Autodesk Inventor part; units mm, degrees
(part 2 of 2)
  spline S254 degree 2 poles (134.5802, -22.8415) (134.5802, -22.7633) (134.5214, -22.7045) (134.4921, -22.7045) knots 0 0 0 1 2 2 2
  spline S255 degree 2 poles (123.7465, -14.2784) (123.7074, -14.2784) (123.6487, -14.3273) (123.6487, -14.4154) knots 0 0 0 1 2 2 2
  line L195 (123.6487, -14.4154) -> (123.6487, -16.6761)
  spline S256 degree 2 poles (123.6487, -16.6761) (123.6487, -16.7544) (123.7074, -16.8229) (123.7465, -16.8229) knots 0 0 0 1 2 2 2
  spline S257 degree 2 poles (123.7465, -16.8229) (123.7759, -16.8229) (123.8346, -16.7641) (123.8346, -16.6761) knots 0 0 0 1 2 2 2
  line L196 (123.8346, -16.6761) -> (123.8346, -16.5391)
  spline S258 degree 2 poles (123.8346, -16.5391) (123.8248, -16.1476) (124.5001, -15.6191) (126.0855, -15.3647) (127.4458, -15.3647) knots 0 0 0 1 2 3 3 3
  line L197 (127.4458, -15.3647) -> (131.5366, -15.3647)
  spline S259 degree 2 poles (131.5366, -15.3647) (132.9262, -15.3451) (134.4627, -16.2944) (134.4725, -17.4981) knots 0 0 0 1 2 2 2
  spline S260 degree 2 poles (134.4725, -17.4981) (134.4529, -18.3398) (133.3764, -19.1325) (132.5054, -19.1227) knots 0 0 0 1 2 2 2
  line L198 (132.5054, -19.1227) -> (124.4414, -19.1227)
  spline S261 degree 2 poles (124.4414, -19.1227) (124.0695, -19.1325) (123.8248, -19.0738) (123.8346, -18.9661) knots 0 0 0 1 2 2 2
  line L199 (123.8346, -18.9661) -> (123.8346, -18.5061)
  spline S262 degree 2 poles (123.8346, -18.5061) (123.8346, -18.4181) (123.7759, -18.3593) (123.7465, -18.3691) knots 0 0 0 1 2 2 2
  spline S263 degree 2 poles (123.7465, -18.3691) (123.7074, -18.3691) (123.6487, -18.4278) (123.6487, -18.5061) knots 0 0 0 1 2 2 2
  line L200 (123.6487, -18.5061) -> (123.6487, -22.0391)
  spline S264 degree 2 poles (123.6487, -22.0391) (123.6487, -22.1173) (123.7074, -22.1761) (123.7465, -22.1761) knots 0 0 0 1 2 2 2
  spline S265 degree 2 poles (123.7465, -22.1761) (123.7759, -22.1761) (123.8346, -22.1173) (123.8346, -22.0391) knots 0 0 0 1 2 2 2
  line L201 (123.8346, -22.0391) -> (123.8346, -21.5987)
  spline S266 degree 2 poles (123.8346, -21.5987) (123.8248, -21.5008) (124.0695, -21.4323) (124.4414, -21.4323) knots 0 0 0 1 2 2 2
  line L202 (124.4414, -21.4323) -> (132.0944, -21.4323)
  spline S267 degree 2 poles (132.0944, -21.4323) (132.8088, -21.4323) (134.0223, -20.6787) (134.7563, -19.2206) (134.7661, -18.1538) knots 0 0 0 1 2 3 3 3
  spline S268 degree 2 poles (134.7661, -18.1538) (134.7759, -17.1556) (134.2083, -15.8246) (132.8382, -15.1592) (131.6442, -15.1592) knots 0 0 0 1 2 3 3 3
  line L203 (131.6442, -15.1592) -> (127.3382, -15.1592)
  spline S269 degree 2 poles (127.3382, -15.1592) (125.9778, -15.1592) (124.4414, -15.0222) (123.8248, -14.709) (123.8346, -14.4448) knots 0 0 0 1 2 3 3 3
  line L204 (123.8346, -14.4448) -> (123.8346, -14.4154)
  spline S270 degree 2 poles (123.8346, -14.4154) (123.8346, -14.3273) (123.7759, -14.2784) (123.7465, -14.2784) knots 0 0 0 1 2 2 2
  spline S271 degree 2 poles (134.4921, -4.4625) (134.4529, -4.4528) (134.3942, -4.5115) (134.3942, -4.5996) knots 0 0 0 1 2 2 2
  line L205 (134.3942, -4.5996) -> (134.3942, -5.0302)
  spline S272 degree 2 poles (134.3942, -5.0302) (134.404, -5.1378) (134.1691, -5.1867) (133.7972, -5.1867) knots 0 0 0 1 2 2 2
  line L206 (133.7972, -5.1867) -> (124.4414, -5.1867)
  spline S273 degree 2 poles (124.4414, -5.1867) (124.0695, -5.1867) (123.8248, -5.1378) (123.8346, -5.0302) knots 0 0 0 1 2 2 2
  line L207 (123.8346, -5.0302) -> (123.8346, -4.5996)
  spline S274 degree 2 poles (123.8346, -4.5996) (123.8346, -4.5115) (123.7759, -4.4528) (123.7465, -4.4625) knots 0 0 0 1 2 2 2
  spline S275 degree 2 poles (123.7465, -4.4625) (123.7074, -4.4625) (123.6487, -4.5213) (123.6487, -4.5996) knots 0 0 0 1 2 2 2
  line L208 (123.6487, -4.5996) -> (123.6487, -7.4866)
  spline S276 degree 2 poles (123.6487, -7.4866) (123.6487, -7.5746) (123.7172, -7.6431) (123.7759, -7.6431) knots 0 0 0 1 2 2 2
  line L209 (123.7759, -7.6431) -> (131.9182, -9.0035)
  line L210 (131.9182, -9.0035) -> (131.9182, -9.023)
  line L211 (131.9182, -9.023) -> (123.7759, -10.5497)
  spline S277 degree 2 poles (123.7759, -10.5497) (123.7172, -10.5693) (123.6487, -10.6574) (123.6487, -10.7259) knots 0 0 0 1 2 2 2
  line L212 (123.6487, -10.7259) -> (123.6487, -13.7303)
  spline S278 degree 2 poles (123.6487, -13.7303) (123.6487, -13.8086) (123.7074, -13.8576) (123.7465, -13.8478) knots 0 0 0 1 2 2 2
  spline S279 degree 2 poles (123.7465, -13.8478) (123.7759, -13.8576) (123.8346, -13.8086) (123.8346, -13.7303) knots 0 0 0 1 2 2 2
  line L213 (123.8346, -13.7303) -> (123.8346, -13.2312)
  spline S280 degree 2 poles (123.8346, -13.2312) (123.8248, -13.1334) (124.0695, -13.0746) (124.4414, -13.0746) knots 0 0 0 1 2 2 2
  line L214 (124.4414, -13.0746) -> (130.9004, -13.0746)
  spline S281 degree 2 poles (130.9004, -13.0746) (132.2608, -13.0746) (133.7972, -13.2117) (134.404, -13.5248) (134.3942, -13.7891) knots 0 0 0 1 2 3 3 3
  line L215 (134.3942, -13.7891) -> (134.3942, -13.8184)
  spline S282 degree 2 poles (134.3942, -13.8184) (134.3942, -13.9065) (134.4529, -13.9652) (134.4921, -13.9554) knots 0 0 0 1 2 2 2
  spline S283 degree 2 poles (134.4921, -13.9554) (134.5214, -13.9652) (134.5802, -13.8967) (134.5802, -13.8184) knots 0 0 0 1 2 2 2
  line L216 (134.5802, -13.8184) -> (134.5802, -11.7045)
  spline S284 degree 2 poles (134.5802, -11.7045) (134.5802, -11.6165) (134.5214, -11.5773) (134.4921, -11.5773) knots 0 0 0 1 2 2 2
  spline S285 degree 2 poles (134.4921, -11.5773) (134.4529, -11.5773) (134.3942, -11.6165) (134.3942, -11.7045) knots 0 0 0 1 2 2 2
  line L217 (134.3942, -11.7045) -> (134.3942, -11.8122)
  spline S286 degree 2 poles (134.3942, -11.8122) (134.404, -12.1645) (133.7874, -12.6343) (132.2118, -12.8593) (130.7928, -12.8593) knots 0 0 0 1 2 3 3 3
  line L218 (130.7928, -12.8593) -> (124.2261, -12.8593)
  line L219 (124.2261, -12.8593) -> (124.2261, -12.8496)
  line L220 (124.2261, -12.8496) -> (134.5019, -10.8042)
  spline S287 degree 2 poles (134.5019, -10.8042) (134.5704, -10.7944) (134.6389, -10.7357) (134.6389, -10.6672) knots 0 0 0 1 2 2 2
  line L221 (134.6389, -10.6672) -> (134.6389, -9.346)
  spline S288 degree 2 poles (134.6389, -9.346) (134.6389, -9.2775) (134.5704, -9.1992) (134.4823, -9.1894) knots 0 0 0 1 2 2 2
  line L222 (134.4823, -9.1894) -> (124.2261, -7.5355)
  line L223 (124.2261, -7.5355) -> (124.2261, -7.5061)
  line L224 (124.2261, -7.5061) -> (133.7874, -7.5061)
  spline S289 degree 2 poles (133.7874, -7.5061) (134.1593, -7.5061) (134.404, -7.5551) (134.3942, -7.6627) knots 0 0 0 1 2 2 2
  line L225 (134.3942, -7.6627) -> (134.3942, -8.0933)
  spline S290 degree 2 poles (134.3942, -8.0933) (134.3942, -8.1716) (134.4529, -8.2303) (134.4823, -8.2303) knots 0 0 0 1 2 2 2
  spline S291 degree 2 poles (134.4823, -8.2303) (134.5214, -8.2303) (134.5802, -8.1716) (134.5802, -8.0933) knots 0 0 0 1 2 2 2
  line L226 (134.5802, -8.0933) -> (134.5802, -4.5996)
  spline S292 degree 2 poles (134.5802, -4.5996) (134.5802, -4.5213) (134.5214, -4.4625) (134.4921, -4.4625) knots 0 0 0 1 2 2 2
  line L227 (137.0494, -38.9843) -> (137.0494, -40.7972)
  line L228 (137.0494, -40.7972) -> (136.8853, -40.7972)
  spline S293 degree 2 poles (136.8853, -40.7972) (136.7138, -40.7972) (136.481, -40.6747) (136.4247, -40.5497) knots 0 0 0 1 2 2 2
  spline S294 degree 2 poles (136.4247, -40.5497) (136.388, -40.4689) (136.3463, -40.1504) (136.3463, -39.952) knots 0 0 0 1 2 2 2
  line L229 (136.3463, -39.952) -> (136.3463, -38.9843)
  line L230 (136.3463, -38.9843) -> (135.8024, -38.9843)
  line L231 (135.8024, -38.9843) -> (135.8024, -40.0353)
  spline S295 degree 2 poles (135.8024, -40.0353) (135.8024, -40.1847) (135.8098, -40.3758) (135.8294, -40.5228) (135.849, -40.6061) knots 0 0 0 1 2 3 3 3
  spline S296 degree 2 poles (135.849, -40.6061) (135.9029, -40.8658) (136.1797, -41.2332) (136.3929, -41.3312) knots 0 0 0 1 2 2 2
  spline S297 degree 2 poles (136.3929, -41.3312) (136.5153, -41.3876) (136.9637, -41.4464) (137.2601, -41.4464) knots 0 0 0 1 2 2 2
  line L232 (137.2601, -41.4464) -> (138.85, -41.4464)
  line L233 (138.85, -41.4464) -> (138.85, -40.7972)
  line L234 (138.85, -40.7972) -> (137.5933, -40.7972)
  line L235 (137.5933, -40.7972) -> (137.5933, -38.9843)
  line L236 (137.5933, -38.9843) -> (137.0494, -38.9843)
  spline S298 degree 2 poles (135.7804, -37.1568) (135.7804, -37.4899) (135.9323, -38.0314) (136.0768, -38.2126) knots 0 0 0 1 2 2 2
  spline S299 degree 2 poles (136.0768, -38.2126) (136.2581, -38.438) (136.9, -38.6732) (137.3385, -38.6732) knots 0 0 0 1 2 2 2
  spline S300 degree 2 poles (137.3385, -38.6732) (137.6447, -38.6732) (138.1445, -38.5409) (138.3331, -38.4086) knots 0 0 0 1 2 2 2
  spline S301 degree 2 poles (138.3331, -38.4086) (138.5903, -38.2273) (138.8647, -37.5659) (138.8671, -37.1249) knots 0 0 0 1 2 2 2
  spline S302 degree 2 poles (138.8671, -37.1249) (138.8647, -36.4047) (138.1028, -35.6697) (137.3556, -35.6673) knots 0 0 0 1 2 2 2
  spline S303 degree 2 poles (137.3556, -35.6673) (137.0102, -35.6673) (136.4369, -35.8241) (136.2508, -35.9637) knots 0 0 0 1 2 2 2
  spline S304 degree 2 poles (136.2508, -35.9637) (136.0278, -36.1377) (135.7829, -36.7575) (135.7804, -37.1568) knots 0 0 0 1 2 2 2
  spline S305 degree 2 poles (136.2973, -37.1739) (136.2949, -36.7648) (136.7897, -36.3777) (137.314, -36.3802) knots 0 0 0 1 2 2 2
  spline S306 degree 2 poles (137.314, -36.3802) (137.8505, -36.3777) (138.3576, -36.7599) (138.3551, -37.1666) knots 0 0 0 1 2 2 2
  spline S307 degree 2 poles (138.3551, -37.1666) (138.3576, -37.5757) (137.8505, -37.9628) (137.3189, -37.9603) knots 0 0 0 1 2 2 2
  spline S308 degree 2 poles (137.3189, -37.9603) (137.0763, -37.9603) (136.7162, -37.8917) (136.6035, -37.8182) knots 0 0 0 1 2 2 2
  spline S309 degree 2 poles (136.6035, -37.8182) (136.4541, -37.7251) (136.2973, -37.392) (136.2973, -37.1739) knots 0 0 0 1 2 2 2
  line L237 (135.8024, -34.5894) -> (135.8024, -35.2386)
  line L238 (135.8024, -35.2386) -> (137.6422, -35.2386)
  spline S310 degree 2 poles (137.6422, -35.2386) (137.8725, -35.2386) (138.1984, -35.1871) (138.4384, -35.0646) (138.5438, -34.9593) knots 0 0 0 1 2 3 3 3
  spline S311 degree 2 poles (138.5438, -34.9593) (138.7079, -34.7952) (138.872, -34.2758) (138.872, -33.9108) knots 0 0 0 1 2 2 2
  spline S312 degree 2 poles (138.872, -33.9108) (138.872, -33.5825) (138.7251, -33.0901) (138.5756, -32.9088) knots 0 0 0 1 2 2 2
  spline S313 degree 2 poles (138.5756, -32.9088) (138.4335, -32.7398) (137.9607, -32.5805) (137.5982, -32.5805) knots 0 0 0 1 2 2 2
  line L239 (137.5982, -32.5805) -> (135.8024, -32.5805)
  line L240 (135.8024, -32.5805) -> (135.8024, -33.2297)
  line L241 (135.8024, -33.2297) -> (137.63, -33.2297)
  spline S314 degree 2 poles (137.63, -33.2297) (137.7917, -33.2297) (138.0048, -33.2567) (138.0685, -33.2836) knots 0 0 0 1 2 2 2
  spline S315 degree 2 poles (138.0685, -33.2836) (138.2057, -33.3498) (138.36, -33.6707) (138.36, -33.8961) knots 0 0 0 1 2 2 2
  spline S316 degree 2 poles (138.36, -33.8961) (138.36, -34.0529) (138.2669, -34.3297) (138.1861, -34.4203) knots 0 0 0 1 2 2 2
  spline S317 degree 2 poles (138.1861, -34.4203) (138.1053, -34.511) (137.848, -34.5894) (137.63, -34.5894) knots 0 0 0 1 2 2 2
  line L242 (137.63, -34.5894) -> (135.8024, -34.5894)
  line L243 (137.6937, -31.3458) -> (137.6937, -30.8265)
  spline S318 degree 2 poles (137.6937, -30.8265) (137.6912, -30.5399) (137.8235, -30.1969) (138.142, -30.0254) (138.4164, -29.9985) knots 0 0 0 1 2 3 3 3
  spline S319 degree 2 poles (138.4164, -29.9985) (138.4654, -29.996) (138.6222, -29.9789) (138.6859, -29.9715) knots 0 0 0 1 2 2 2
  spline S320 degree 2 poles (138.6859, -29.9715) (138.7349, -29.9642) (138.801, -29.9519) (138.85, -29.9348) knots 0 0 0 1 2 2 2
  line L244 (138.85, -29.9348) -> (138.85, -29.2072)
  spline S321 degree 2 poles (138.85, -29.2072) (138.7961, -29.2292) (138.6908, -29.2513) (138.5291, -29.2709) (138.3894, -29.2807) knots 0 0 0 1 2 3 3 3
  spline S322 degree 2 poles (138.3894, -29.2807) (138.0318, -29.2978) (137.6129, -29.5673) (137.5418, -29.8343) knots 0 0 0 1 2 2 2
  spline S323 degree 2 poles (137.5418, -29.8343) (137.4414, -29.5403) (137.0004, -29.2537) (136.6525, -29.2537) knots 0 0 0 1 2 2 2
  spline S324 degree 2 poles (136.6525, -29.2537) (136.4418, -29.2537) (136.0915, -29.4301) (135.9813, -29.5918) knots 0 0 0 1 2 2 2
  spline S325 degree 2 poles (135.9813, -29.5918) (135.8857, -29.7265) (135.8024, -30.1626) (135.8024, -30.5056) knots 0 0 0 1 2 2 2
  line L245 (135.8024, -30.5056) -> (135.8024, -31.995)
  line L246 (135.8024, -31.995) -> (138.85, -31.995)
  line L247 (138.85, -31.995) -> (138.85, -31.3458)
  line L248 (138.85, -31.3458) -> (137.6937, -31.3458)
  line L249 (137.1498, -31.3458) -> (136.3463, -31.3458)
  line L250 (136.3463, -31.3458) -> (136.3463, -30.437)
  spline S326 degree 2 poles (136.3463, -30.437) (136.3463, -30.3537) (136.3586, -30.2336) (136.3684, -30.1944) knots 0 0 0 1 2 2 2
  spline S327 degree 2 poles (136.3684, -30.1944) (136.4076, -30.0891) (136.5913, -29.9715) (136.7309, -29.9715) knots 0 0 0 1 2 2 2
  spline S328 degree 2 poles (136.7309, -29.9715) (136.9514, -29.9691) (137.1523, -30.1895) (137.1498, -30.437) knots 0 0 0 1 2 2 2
  line L251 (137.1498, -30.437) -> (137.1498, -31.3458)
  line L252 (136.3463, -28.0435) -> (138.85, -28.0435)
  line L253 (138.85, -28.0435) -> (138.85, -27.3943)
  line L254 (138.85, -27.3943) -> (136.3463, -27.3943)
  line L255 (136.3463, -27.3943) -> (136.3463, -26.3899)
  line L256 (136.3463, -26.3899) -> (135.8024, -26.3899)
  line L257 (135.8024, -26.3899) -> (135.8024, -29.0161)
  line L258 (135.8024, -29.0161) -> (136.3463, -29.0161)
  line L259 (136.3463, -29.0161) -> (136.3463, -28.0435)
  line L260 (135.8024, -23.5849) -> (135.8024, -24.2341)
  line L261 (135.8024, -24.2341) -> (137.0494, -24.2341)
  line L262 (137.0494, -24.2341) -> (137.0494, -25.4075)
  line L263 (137.0494, -25.4075) -> (135.8024, -25.4075)
  line L264 (135.8024, -25.4075) -> (135.8024, -26.0567)
  line L265 (135.8024, -26.0567) -> (138.85, -26.0567)
  line L266 (138.85, -26.0567) -> (138.85, -25.4075)
  line L267 (138.85, -25.4075) -> (137.5933, -25.4075)
  line L268 (137.5933, -25.4075) -> (137.5933, -24.2341)
  line L269 (137.5933, -24.2341) -> (138.85, -24.2341)
  line L270 (138.85, -24.2341) -> (138.85, -23.5849)
  line L271 (138.85, -23.5849) -> (135.8024, -23.5849)
  line L272 (135.8024, -19.5378) -> (135.8024, -20.6329)
  spline S329 degree 2 poles (135.8024, -20.6329) (135.8024, -20.8362) (135.849, -21.1326) (135.9592, -21.3629) (136.0499, -21.4707) knots 0 0 0 1 2 3 3 3
  spline S330 degree 2 poles (136.0499, -21.4707) (136.2655, -21.723) (136.9, -21.9852) (137.3066, -21.9852) knots 0 0 0 1 2 2 2
  spline S331 degree 2 poles (137.3066, -21.9852) (137.6888, -21.9852) (138.3037, -21.7794) (138.507, -21.5834) knots 0 0 0 1 2 2 2
  spline S332 degree 2 poles (138.507, -21.5834) (138.6344, -21.4658) (138.7863, -21.1522) (138.85, -20.7039) (138.85, -20.383) knots 0 0 0 1 2 3 3 3
  line L273 (138.85, -20.383) -> (138.85, -19.5378)
  line L274 (138.85, -19.5378) -> (138.3061, -19.5378)
  line L275 (138.3061, -19.5378) -> (138.3061, -20.3536)
  spline S333 degree 2 poles (138.3061, -20.3536) (138.3086, -20.6623) (138.1739, -21.042) (137.8676, -21.2282) (137.608, -21.2502) knots 0 0 0 1 2 3 3 3
  line L276 (137.608, -21.2502) -> (137.608, -19.5378)
  line L277 (137.608, -19.5378) -> (137.0641, -19.5378)
  line L278 (137.0641, -19.5378) -> (137.0641, -21.2502)
  spline S334 degree 2 poles (137.0641, -21.2502) (136.9171, -21.2404) (136.7432, -21.2135) (136.6305, -21.162) (136.5692, -21.1179) knots 0 0 0 1 2 3 3 3
  spline S335 degree 2 poles (136.5692, -21.1179) (136.4835, -21.0542) (136.3855, -20.8779) (136.3463, -20.5986) (136.3463, -20.383) knots 0 0 0 1 2 3 3 3
  line L279 (136.3463, -20.383) -> (136.3463, -19.5378)
  line L280 (136.3463, -19.5378) -> (135.8024, -19.5378)
  line L281 (135.8024, -19.0258) -> (138.85, -19.0258)
  line L282 (138.85, -19.0258) -> (138.85, -17.7323)
  spline S336 degree 2 poles (138.85, -17.7323) (138.85, -17.5314) (138.8378, -17.2595) (138.8084, -17.066) (138.7814, -16.9827) knots 0 0 0 1 2 3 3 3
  spline S337 degree 2 poles (138.7814, -16.9827) (138.7079, -16.7377) (138.3943, -16.4192) (138.142, -16.3335) knots 0 0 0 1 2 2 2
  spline S338 degree 2 poles (138.142, -16.3335) (137.9681, -16.2747) (137.5369, -16.2061) (137.3336, -16.2061) knots 0 0 0 1 2 2 2
  spline S339 degree 2 poles (137.3336, -16.2061) (137.1082, -16.2061) (136.6819, -16.282) (136.3341, -16.4168) (136.2238, -16.5074) knots 0 0 0 1 2 3 3 3
  spline S340 degree 2 poles (136.2238, -16.5074) (136.0009, -16.6813) (135.8, -17.2644) (135.8024, -17.7323) knots 0 0 0 1 2 2 2
  line L283 (135.8024, -17.7323) -> (135.8024, -19.0258)
  line L284 (136.3463, -18.3766) -> (136.3463, -17.7323)
  spline S341 degree 2 poles (136.3463, -17.7323) (136.3463, -17.5388) (136.4124, -17.2865) (136.4884, -17.1983) knots 0 0 0 1 2 2 2
  spline S342 degree 2 poles (136.4884, -17.1983) (136.5986, -17.0684) (137.0469, -16.9214) (137.3287, -16.919) knots 0 0 0 1 2 2 2
  spline S343 degree 2 poles (137.3287, -16.919) (137.5688, -16.919) (137.9803, -17.0317) (138.1053, -17.1297) knots 0 0 0 1 2 2 2
  spline S344 degree 2 poles (138.1053, -17.1297) (138.2057, -17.213) (138.3061, -17.5192) (138.3061, -17.7323) knots 0 0 0 1 2 2 2
  line L285 (138.3061, -17.7323) -> (138.3061, -18.3766)
  line L286 (138.3061, -18.3766) -> (136.3463, -18.3766)
  line L287 (138.85, -15.7504) -> (138.85, -15.1012)
  line L288 (138.85, -15.1012) -> (135.8024, -15.1012)
  line L289 (135.8024, -15.1012) -> (135.8024, -15.7504)
  line L290 (135.8024, -15.7504) -> (138.85, -15.7504)
  line L291 (136.3463, -13.7955) -> (138.85, -13.7955)
  line L292 (138.85, -13.7955) -> (138.85, -13.1463)
  line L293 (138.85, -13.1463) -> (136.3463, -13.1463)
  line L294 (136.3463, -13.1463) -> (136.3463, -12.1419)
  line L295 (136.3463, -12.1419) -> (135.8024, -12.1419)
  line L296 (135.8024, -12.1419) -> (135.8024, -14.7681)
  line L297 (135.8024, -14.7681) -> (136.3463, -14.7681)
  line L298 (136.3463, -14.7681) -> (136.3463, -13.7955)
  line L299 (138.85, -11.8087) -> (138.85, -11.1595)
  line L300 (138.85, -11.1595) -> (135.8024, -11.1595)
  line L301 (135.8024, -11.1595) -> (135.8024, -11.8087)
  line L302 (135.8024, -11.8087) -> (138.85, -11.8087)
  spline S345 degree 2 poles (135.7804, -9.1874) (135.7804, -9.5206) (135.9323, -10.062) (136.0768, -10.2433) knots 0 0 0 1 2 2 2
  spline S346 degree 2 poles (136.0768, -10.2433) (136.2581, -10.4687) (136.9, -10.7038) (137.3385, -10.7038) knots 0 0 0 1 2 2 2
  spline S347 degree 2 poles (137.3385, -10.7038) (137.6447, -10.7038) (138.1445, -10.5716) (138.3331, -10.4393) knots 0 0 0 1 2 2 2
  spline S348 degree 2 poles (138.3331, -10.4393) (138.5903, -10.258) (138.8647, -9.5965) (138.8671, -9.1556) knots 0 0 0 1 2 2 2
  spline S349 degree 2 poles (138.8671, -9.1556) (138.8647, -8.4353) (138.1028, -7.7004) (137.3556, -7.6979) knots 0 0 0 1 2 2 2
  spline S350 degree 2 poles (137.3556, -7.6979) (137.0102, -7.6979) (136.4369, -7.8547) (136.2508, -7.9944) knots 0 0 0 1 2 2 2
  spline S351 degree 2 poles (136.2508, -7.9944) (136.0278, -8.1683) (135.7829, -8.7881) (135.7804, -9.1874) knots 0 0 0 1 2 2 2
  spline S352 degree 2 poles (136.2973, -9.2046) (136.2949, -8.7954) (136.7897, -8.4084) (137.314, -8.4108) knots 0 0 0 1 2 2 2
  spline S353 degree 2 poles (137.314, -8.4108) (137.8505, -8.4084) (138.3576, -8.7905) (138.3551, -9.1972) knots 0 0 0 1 2 2 2
  spline S354 degree 2 poles (138.3551, -9.1972) (138.3576, -9.6063) (137.8505, -9.9934) (137.3189, -9.9909) knots 0 0 0 1 2 2 2
  spline S355 degree 2 poles (137.3189, -9.9909) (137.0763, -9.9909) (136.7162, -9.9224) (136.6035, -9.8489) knots 0 0 0 1 2 2 2
  spline S356 degree 2 poles (136.6035, -9.8489) (136.4541, -9.7558) (136.2973, -9.4226) (136.2973, -9.2046) knots 0 0 0 1 2 2 2
  line L303 (136.6158, -6.62) -> (138.85, -5.3755)
  line L304 (138.85, -5.3755) -> (138.85, -4.5793)
  line L305 (138.85, -4.5793) -> (135.8024, -4.5793)
  line L306 (135.8024, -4.5793) -> (135.8024, -5.1967)
  line L307 (135.8024, -5.1967) -> (138.0734, -5.1967)
  line L308 (138.0734, -5.1967) -> (135.8024, -6.4093)
  line L309 (135.8024, -6.4093) -> (135.8024, -7.2374)
  line L310 (135.8024, -7.2374) -> (138.85, -7.2374)
  line L311 (138.85, -7.2374) -> (138.85, -6.62)
  line L312 (138.85, -6.62) -> (136.6158, -6.62)
  point P0 (70.425, -34.6)
  dimension "d27" = 25
  dimension "d28" = 2
  constraints: 4 end point, 4 point on line, 3 vertical, 1 perpendicular
  measures "d27" distance between parallel lines of L2 L11
  measures "d28" distance between parallel lines of L2 L14
emboss "Emboss2" sketch "Sketch4" operation cut depth 0.5 direction (0, -1, 0) contours S15 S14 L26 S13 L25 S12 L24 S11 L23 S10 S9 L22 S8 S7 L21 S6 L20 S5 L19 S4 L18 S3 S2 L17 S1 L16 S0 L15 | S37 L48 S36 L47 S35 L46 S34 L45 L44 L43 S33 L42 S32 L41 S31 L40 S30 S29 L39 S28 S27 L38 S26 L37 L36 L35 S25 L34 S24 S23 L33 S22 S21 L32 S20 L31 L30 L29 S19 L28 S18 S17 L27 S16 | S49 L56 S48 S47 L55 S46 L54 S45 L53 S44 S43 L52 S42 S41 L51 S40 L50 S39 L49 S38 | S63 L66 S62 S61 L65 S60 L64 S59 L63 S58 S57 L62 S56 S55 L61 S54 L60 S53 L59 S52 L58 S51 S50 L57 | S75 L74 S74 S73 L73 S72 L72 S71 L71 S70 S69 L70 S68 S67 L69 S66 L68 S65 L67 S64 | S98 L83 S97 L82 S96 S95 L81 S94 S93 S92 S91 S90 S89 L80 S88 S87 L79 S86 S85 L78 S84 S83 S82 S81 S80 L77 S79 L76 S78 S77 L75 S76 | S126 L103 S125 S124 L102 S123 L101 S122 L100 S121 L99 S120 L98 S119 S118 L97 S117 S116 L96 S115 L95 S114 L94 S113 S112 L93 S111 S110 L92 S109 L91 S108 L90 S107 L89 S106 L88 S105 S104 L87 S103 S102 L86 S101 L85 S100 L84 S99 | S142 S141 L115 S140 L114 S139 L113 S138 L112 S137 S136 L111 S135 S134 L110 S133 L109 S132 L108 S131 L107 S130 S129 L106 S128 L105 S127 L104 | S154 L123 S153 S152 L122 S151 L121 S150 L120 S149 S148 L119 S147 S146 L118 S145 L117 S144 L116 S143 | S176 L145 S175 S174 L144 S173 L143 L142 L141 S172 L140 S171 L139 L138 L137 S170 L136 S169 S168 L135 S167 S166 L134 S165 L133 S164 L132 S163 S162 L131 S161 L130 L129 L128 S160 L127 S159 S158 L126 S157 L125 S156 L124 S155 | S188 L153 S187 L152 S186 L151 S185 S184 L150 S183 S182 L149 S181 L148 S180 L147 S179 S178 L146 S177 | S216 L174 S215 S214 L173 S213 L172 S212 L171 S211 S210 L170 S209 L169 S208 S207 L168 S206 L167 S205 L166 S204 L165 S203 L164 S202 S201 L163 S200 S199 L162 S198 L161 S197 L160 S196 L159 S195 L158 S194 S193 L157 | S238 S237 S236 S235 S234 L183 S233 L182 S232 L181 S231 S230 L180 S229 S228 L179 S227 L178 S226 L177 S225 S224 L176 S223 S222 L175 S221 S220 S219 S218 S217 | S254 L194 S253 S252 L193 S251 L192 S250 L191 S249 S248 L190 S247 S246 L189 S245 L188 S244 L187 S243 | S270 L204 S269 L203 S268 S267 L202 S266 L201 S265 S264 L200 S263 S262 L199 S261 L198 S260 S259 L197 S258 L196 S257 S256 L195 S255 | S292 L226 S291 S290 L225 S289 L224 L223 L222 S288 L221 S287 L220 L219 L218 S286 L217 S285 S284 L216 S283 S282 L215 S281 L214 S280 L213 S279 S278 L212 S277 L211 L210 L209 S276 L208 S275 S274 L207 S273 L206 S272 L205 S271 | L236 L235 L234 L233 L232 S297 S296 S295 L231 L230 L229 S294 S293 L228 L227 | S304 S303 S302 S301 S300 S299 S298 | L242 S317 S316 S315 S314 L241 L240 L239 S313 S312 S311 S310 L238 L237 | L248 L247 L246 L245 S325 S324 S323 S322 S321 L244 S320 S319 S318 L243 | L259 L258 L257 L256 L255 L254 L253 L252 | L271 L270 L269 L268 L267 L266 L265 L264 L263 L262 L261 L260 | L280 L279 S335 S334 L278 L277 L276 S333 L275 L274 L273 S332 S331 S330 S329 L272 | L283 S340 S339 S338 S337 S336 L282 L281 | L290 L289 L288 L287 | L298 L297 L296 L295 L294 L293 L292 L291 | L302 L301 L300 L299 | S351 S350 S349 S348 S347 S346 S345 | L312 L311 L310 L309 L308 L307 L306 L305 L304 L303
sketch "Sketch6" plane through (-70.425, 1, -34.6) normal (0, 1, 0) x (1, 0, 0)
  line L0 (47.5966, -31.7925) -> (52.4593, -28.985)
  line L1 (52.4593, -28.985) -> (57.322, -31.7925)
  line L2 (57.322, -31.7925) -> (57.322, -37.4075)
  line L3 (57.322, -37.4075) -> (52.4593, -40.215)
  line L4 (52.4593, -40.215) -> (47.5966, -37.4075)
  line L5 (47.5966, -37.4075) -> (47.5966, -31.7925)
  line L6 (50.0279, -38.8112) -> (54.8906, -30.3888) construction
  line L7 (42.1338, -41.2542) -> (46.9966, -38.4467)
  line L8 (46.9966, -38.4467) -> (51.8593, -41.2542)
  line L9 (51.8593, -41.2542) -> (51.8593, -46.8692)
  line L10 (51.8593, -46.8692) -> (46.9966, -49.6766)
  line L11 (46.9966, -49.6766) -> (42.1338, -46.8692)
  line L12 (42.1338, -46.8692) -> (42.1338, -41.2542)
  line L13 (36.6711, -56.3308) -> (36.6711, -50.7159)
  line L14 (36.6711, -50.7159) -> (41.5338, -47.9084)
  line L15 (41.5338, -47.9084) -> (46.3966, -50.7159)
  line L16 (46.3966, -50.7159) -> (46.3966, -56.3308)
  line L17 (46.3966, -56.3308) -> (41.5338, -59.1383)
  line L18 (41.5338, -59.1383) -> (36.6711, -56.3308)
  line L19 (31.2084, -60.1776) -> (36.0711, -57.3701)
  line L20 (36.0711, -57.3701) -> (40.9338, -60.1776)
  line L21 (40.9338, -60.1776) -> (40.9338, -65.7925)
  line L22 (40.9338, -65.7925) -> (36.0711, -68.6)
  line L23 (36.0711, -68.6) -> (31.2084, -65.7925)
  line L24 (31.2084, -65.7925) -> (31.2084, -60.1776)
  line L25 (0, -69.2) -> (0, 0) projected
  line L26 (104.9185, -32.4225) -> (104.9185, -28.9287) projected
  line L27 (0, -34.6) -> (104.9185, -34.6) construction
  line L28 (40.9338, -46.8692) -> (36.0711, -49.6766)
  line L29 (36.0711, -49.6766) -> (31.2084, -46.8692)
  line L30 (31.2084, -46.8692) -> (31.2084, -41.2542)
  line L31 (31.2084, -41.2542) -> (36.0711, -38.4467)
  line L32 (36.0711, -38.4467) -> (40.9338, -41.2542)
  line L33 (40.9338, -41.2542) -> (40.9338, -46.8692)
  line L34 (35.4711, -56.3308) -> (30.6084, -59.1383)
  line L35 (30.6084, -59.1383) -> (25.7457, -56.3308)
  line L36 (25.7457, -56.3308) -> (25.7457, -50.7159)
  line L37 (25.7457, -50.7159) -> (30.6084, -47.9084)
  line L38 (30.6084, -47.9084) -> (35.4711, -50.7159)
  line L39 (35.4711, -50.7159) -> (35.4711, -56.3308)
  line L40 (30.0084, -46.8692) -> (25.1457, -49.6766)
  line L41 (25.1457, -49.6766) -> (20.283, -46.8692)
  line L42 (20.283, -46.8692) -> (20.283, -41.2542)
  line L43 (20.283, -41.2542) -> (25.1457, -38.4467)
  line L44 (25.1457, -38.4467) -> (30.0084, -41.2542)
  line L45 (30.0084, -41.2542) -> (30.0084, -46.8692)
  line L46 (53.0593, -46.8692) -> (53.0593, -41.2542)
  line L47 (47.5966, -50.7159) -> (52.4593, -47.9084)
  line L48 (47.5966, -56.3308) -> (47.5966, -50.7159)
  line L49 (53.0593, -41.2542) -> (57.922, -38.4467)
  line L50 (52.4593, -47.9084) -> (57.322, -50.7159)
  line L51 (57.922, -49.6766) -> (53.0593, -46.8692)
  line L52 (57.922, -38.4467) -> (62.7847, -41.2542)
  line L53 (62.7847, -41.2542) -> (62.7847, -46.8692)
  line L54 (62.7847, -46.8692) -> (57.922, -49.6766)
  line L55 (63.3847, -59.1383) -> (58.522, -56.3308)
  line L56 (57.322, -56.3308) -> (52.4593, -59.1383)
  line L57 (57.322, -50.7159) -> (57.322, -56.3308)
  line L58 (58.522, -56.3308) -> (58.522, -50.7159)
  line L59 (58.522, -50.7159) -> (63.3847, -47.9084)
  line L60 (63.3847, -47.9084) -> (68.2474, -50.7159)
  line L61 (68.2474, -50.7159) -> (68.2474, -56.3308)
  line L62 (68.2474, -56.3308) -> (63.3847, -59.1383)
  line L63 (63.9847, -60.1776) -> (68.8474, -57.3701)
  line L64 (63.9847, -65.7925) -> (63.9847, -60.1776)
  line L65 (68.8474, -57.3701) -> (73.7101, -60.1776)
  line L66 (73.7101, -60.1776) -> (73.7101, -65.7925)
  line L67 (73.7101, -65.7925) -> (68.8474, -68.6)
  line L68 (68.8474, -68.6) -> (63.9847, -65.7925)
  line L69 (52.4593, -59.1383) -> (47.5966, -56.3308)
  line L70 (46.9966, -57.3701) -> (51.8593, -60.1776)
  line L71 (53.0593, -60.1776) -> (57.922, -57.3701)
  line L72 (51.8593, -60.1776) -> (51.8593, -65.7925)
  line L73 (42.1338, -60.1776) -> (46.9966, -57.3701)
  line L74 (53.0593, -65.7925) -> (53.0593, -60.1776)
  line L75 (42.1338, -65.7925) -> (42.1338, -60.1776)
  line L76 (46.9966, -68.6) -> (42.1338, -65.7925)
  line L77 (57.922, -57.3701) -> (62.7847, -60.1776)
  line L78 (62.7847, -60.1776) -> (62.7847, -65.7925)
  line L79 (62.7847, -65.7925) -> (57.922, -68.6)
  line L80 (57.922, -68.6) -> (53.0593, -65.7925)
  line L81 (51.8593, -65.7925) -> (46.9966, -68.6)
  line L82 (63.3847, -40.215) -> (58.522, -37.4075)
  line L83 (63.9847, -46.8692) -> (63.9847, -41.2542)
  line L84 (68.8474, -49.6766) -> (63.9847, -46.8692)
  line L85 (58.522, -37.4075) -> (58.522, -31.7925)
  line L86 (63.9847, -41.2542) -> (68.8474, -38.4467)
  line L87 (68.2474, -37.4075) -> (63.3847, -40.215)
  line L88 (58.522, -31.7925) -> (63.3847, -28.985)
  line L89 (63.3847, -28.985) -> (68.2474, -31.7925)
  line L90 (68.2474, -31.7925) -> (68.2474, -37.4075)
  line L91 (79.1728, -37.4075) -> (74.3101, -40.215)
  line L92 (73.7101, -41.2542) -> (73.7101, -46.8692)
  line L93 (68.8474, -38.4467) -> (73.7101, -41.2542)
  line L94 (74.3101, -40.215) -> (69.4474, -37.4075)
  line L95 (69.4474, -37.4075) -> (69.4474, -31.7925)
  line L96 (69.4474, -31.7925) -> (74.3101, -28.985)
  line L97 (74.3101, -28.985) -> (79.1728, -31.7925)
  line L98 (79.1728, -31.7925) -> (79.1728, -37.4075)
  line L99 (80.3728, -37.4075) -> (80.3728, -31.7925)
  line L100 (85.2355, -40.215) -> (80.3728, -37.4075)
  line L101 (80.3728, -31.7925) -> (85.2355, -28.985)
  line L102 (85.2355, -28.985) -> (90.0982, -31.7925)
  line L103 (90.0982, -31.7925) -> (90.0982, -37.4075)
  line L104 (90.0982, -37.4075) -> (85.2355, -40.215)
  line L105 (73.7101, -46.8692) -> (68.8474, -49.6766)
  line L106 (69.4474, -50.7159) -> (74.3101, -47.9084)
  line L107 (74.9101, -46.8692) -> (74.9101, -41.2542)
  line L108 (74.3101, -47.9084) -> (79.1728, -50.7159)
  line L109 (69.4474, -56.3308) -> (69.4474, -50.7159)
  line L110 (79.7728, -49.6766) -> (74.9101, -46.8692)
  line L111 (74.3101, -59.1383) -> (69.4474, -56.3308)
  line L112 (79.1728, -56.3308) -> (74.3101, -59.1383)
  line L113 (74.9101, -41.2542) -> (79.7728, -38.4467)
  line L114 (79.7728, -38.4467) -> (84.6355, -41.2542)
  line L115 (84.6355, -41.2542) -> (84.6355, -46.8692)
  line L116 (84.6355, -46.8692) -> (79.7728, -49.6766)
  line L117 (79.1728, -50.7159) -> (79.1728, -56.3308)
  line L118 (62.7847, -27.9458) -> (57.922, -30.7533)
  line L119 (68.8474, -30.7533) -> (63.9847, -27.9458)
  line L120 (73.7101, -27.9458) -> (68.8474, -30.7533)
  line L121 (57.922, -30.7533) -> (53.0593, -27.9458)
  line L122 (63.9847, -27.9458) -> (63.9847, -22.3308)
  line L123 (62.7847, -22.3308) -> (62.7847, -27.9458)
  line L124 (53.0593, -27.9458) -> (53.0593, -22.3308)
  line L125 (53.0593, -22.3308) -> (57.922, -19.5234)
  line L126 (57.922, -19.5234) -> (62.7847, -22.3308)
  line L127 (68.2474, -12.8692) -> (68.2474, -18.4841)
  line L128 (68.8474, -19.5234) -> (73.7101, -22.3308)
  line L129 (63.9847, -22.3308) -> (68.8474, -19.5234)
  line L130 (68.2474, -18.4841) -> (63.3847, -21.2916)
  line L131 (63.3847, -21.2916) -> (58.522, -18.4841)
  line L132 (58.522, -18.4841) -> (58.522, -12.8692)
  line L133 (58.522, -12.8692) -> (63.3847, -10.0617)
  line L134 (63.3847, -10.0617) -> (68.2474, -12.8692)
  line L135 (68.8474, -11.8299) -> (63.9847, -9.0224)
  line L136 (73.7101, -9.0224) -> (68.8474, -11.8299)
  line L137 (63.9847, -9.0224) -> (63.9847, -3.4075)
  line L138 (63.9847, -3.4075) -> (68.8474, -0.6)
  line L139 (68.8474, -0.6) -> (73.7101, -3.4075)
  line L140 (73.7101, -3.4075) -> (73.7101, -9.0224)
  line L141 (73.7101, -22.3308) -> (73.7101, -27.9458)
  line L142 (74.9101, -27.9458) -> (74.9101, -22.3308)
  line L143 (74.3101, -21.2916) -> (69.4474, -18.4841)
  line L144 (74.9101, -22.3308) -> (79.7728, -19.5234)
  line L145 (79.7728, -30.7533) -> (74.9101, -27.9458)
  line L146 (79.1728, -18.4841) -> (74.3101, -21.2916)
  line L147 (84.6355, -27.9458) -> (79.7728, -30.7533)
  line L148 (84.6355, -22.3308) -> (84.6355, -27.9458)
  line L149 (69.4474, -18.4841) -> (69.4474, -12.8692)
  line L150 (69.4474, -12.8692) -> (74.3101, -10.0617)
  line L151 (74.3101, -10.0617) -> (79.1728, -12.8692)
  line L152 (79.1728, -12.8692) -> (79.1728, -18.4841)
  line L153 (79.7728, -19.5234) -> (84.6355, -22.3308)
  line L154 (51.8593, -22.3308) -> (51.8593, -27.9458)
  line L155 (57.322, -18.4841) -> (52.4593, -21.2916)
  line L156 (57.322, -12.8692) -> (57.322, -18.4841)
  line L157 (51.8593, -27.9458) -> (46.9966, -30.7533)
  line L158 (52.4593, -21.2916) -> (47.5966, -18.4841)
  line L159 (46.9966, -19.5234) -> (51.8593, -22.3308)
  line L160 (46.9966, -30.7533) -> (42.1338, -27.9458)
  line L161 (42.1338, -27.9458) -> (42.1338, -22.3308)
  line L162 (42.1338, -22.3308) -> (46.9966, -19.5234)
  line L163 (41.5338, -10.0617) -> (46.3966, -12.8692)
  line L164 (47.5966, -12.8692) -> (52.4593, -10.0617)
  line L165 (47.5966, -18.4841) -> (47.5966, -12.8692)
  line L166 (46.3966, -12.8692) -> (46.3966, -18.4841)
  line L167 (46.3966, -18.4841) -> (41.5338, -21.2916)
  line L168 (41.5338, -21.2916) -> (36.6711, -18.4841)
  line L169 (36.6711, -18.4841) -> (36.6711, -12.8692)
  line L170 (36.6711, -12.8692) -> (41.5338, -10.0617)
  line L171 (40.9338, -9.0224) -> (36.0711, -11.8299)
  line L172 (40.9338, -3.4075) -> (40.9338, -9.0224)
  line L173 (36.0711, -11.8299) -> (31.2084, -9.0224)
  line L174 (31.2084, -9.0224) -> (31.2084, -3.4075)
  line L175 (31.2084, -3.4075) -> (36.0711, -0.6)
  line L176 (36.0711, -0.6) -> (40.9338, -3.4075)
  line L177 (52.4593, -10.0617) -> (57.322, -12.8692)
  line L178 (57.922, -11.8299) -> (53.0593, -9.0224)
  line L179 (51.8593, -9.0224) -> (46.9966, -11.8299)
  line L180 (53.0593, -9.0224) -> (53.0593, -3.4075)
  line L181 (62.7847, -9.0224) -> (57.922, -11.8299)
  line L182 (51.8593, -3.4075) -> (51.8593, -9.0224)
  line L183 (62.7847, -3.4075) -> (62.7847, -9.0224)
  line L184 (57.922, -0.6) -> (62.7847, -3.4075)
  line L185 (46.9966, -11.8299) -> (42.1338, -9.0224)
  line L186 (42.1338, -9.0224) -> (42.1338, -3.4075)
  line L187 (42.1338, -3.4075) -> (46.9966, -0.6)
  line L188 (46.9966, -0.6) -> (51.8593, -3.4075)
  line L189 (53.0593, -3.4075) -> (57.922, -0.6)
  line L190 (41.5338, -28.985) -> (46.3966, -31.7925)
  line L191 (40.9338, -22.3308) -> (40.9338, -27.9458)
  line L192 (36.0711, -19.5234) -> (40.9338, -22.3308)
  line L193 (46.3966, -31.7925) -> (46.3966, -37.4075)
  line L194 (40.9338, -27.9458) -> (36.0711, -30.7533)
  line L195 (36.6711, -31.7925) -> (41.5338, -28.985)
  line L196 (46.3966, -37.4075) -> (41.5338, -40.215)
  line L197 (41.5338, -40.215) -> (36.6711, -37.4075)
  line L198 (36.6711, -37.4075) -> (36.6711, -31.7925)
  line L199 (25.7457, -31.7925) -> (30.6084, -28.985)
  line L200 (31.2084, -27.9458) -> (31.2084, -22.3308)
  line L201 (36.0711, -30.7533) -> (31.2084, -27.9458)
  line L202 (30.6084, -28.985) -> (35.4711, -31.7925)
  line L203 (35.4711, -31.7925) -> (35.4711, -37.4075)
  line L204 (35.4711, -37.4075) -> (30.6084, -40.215)
  line L205 (30.6084, -40.215) -> (25.7457, -37.4075)
  line L206 (25.7457, -37.4075) -> (25.7457, -31.7925)
  line L207 (24.5457, -31.7925) -> (24.5457, -37.4075)
  line L208 (19.683, -28.985) -> (24.5457, -31.7925)
  line L209 (24.5457, -37.4075) -> (19.683, -40.215)
  line L210 (19.683, -40.215) -> (14.8203, -37.4075)
  line L211 (14.8203, -37.4075) -> (14.8203, -31.7925)
  line L212 (14.8203, -31.7925) -> (19.683, -28.985)
  line L213 (31.2084, -22.3308) -> (36.0711, -19.5234)
  line L214 (35.4711, -18.4841) -> (30.6084, -21.2916)
  line L215 (30.0084, -22.3308) -> (30.0084, -27.9458)
  line L216 (30.6084, -21.2916) -> (25.7457, -18.4841)
  line L217 (35.4711, -12.8692) -> (35.4711, -18.4841)
  line L218 (25.1457, -19.5234) -> (30.0084, -22.3308)
  line L219 (30.6084, -10.0617) -> (35.4711, -12.8692)
  line L220 (25.7457, -12.8692) -> (30.6084, -10.0617)
  line L221 (30.0084, -27.9458) -> (25.1457, -30.7533)
  line L222 (25.1457, -30.7533) -> (20.283, -27.9458)
  line L223 (20.283, -27.9458) -> (20.283, -22.3308)
  line L224 (20.283, -22.3308) -> (25.1457, -19.5234)
  line L225 (25.7457, -18.4841) -> (25.7457, -12.8692)
  point P0 (70.425, -34.6)
  point P1 (52.4593, -34.6)
  point P2 (46.9966, -44.0617)
  point P3 (41.5338, -53.5234)
  point P4 (36.0711, -62.985)
  point P5 (52.4593, -34.6)
  point P6 (52.4593, -34.6)
  point P7 (36.0711, -44.0617)
  point P8 (30.6084, -53.5234)
  point P9 (25.1457, -44.0617)
  point P10 (52.4593, -53.5234)
  point P11 (54.8906, -38.8112)
  point P12 (57.922, -44.0617)
  point P13 (63.3847, -53.5234)
  point P14 (68.8474, -62.985)
  point P15 (57.922, -62.985)
  point P16 (46.9966, -62.985)
  point P17 (57.322, -31.7925)
  point P18 (57.322, -37.4075)
  point P19 (68.8474, -44.0617)
  point P20 (57.322, -34.6)
  point P21 (63.3847, -34.6)
  point P22 (74.3101, -34.6)
  point P23 (85.2355, -34.6)
  point P24 (79.7728, -44.0617)
  point P25 (74.3101, -53.5234)
  point P26 (52.4593, -28.985)
  point P27 (57.322, -31.7925)
  point P28 (68.8474, -25.1383)
  point P29 (54.8906, -30.3888)
  point P30 (57.922, -25.1383)
  point P31 (63.3847, -15.6766)
  point P32 (68.8474, -6.215)
  point P33 (74.3101, -15.6766)
  point P34 (79.7728, -25.1383)
  point P35 (47.5966, -31.7925)
  point P36 (52.4593, -28.985)
  point P37 (52.4593, -15.6766)
  point P38 (50.0279, -30.3888)
  point P39 (46.9966, -25.1383)
  point P40 (41.5338, -15.6766)
  point P41 (36.0711, -6.215)
  point P42 (46.9966, -6.215)
  point P43 (57.922, -6.215)
  point P44 (47.5966, -37.4075)
  point P45 (47.5966, -31.7925)
  point P46 (36.0711, -25.1383)
  point P47 (47.5966, -34.6)
  point P48 (41.5338, -34.6)
  point P49 (30.6084, -34.6)
  point P50 (19.683, -34.6)
  point P51 (25.1457, -25.1383)
  point P52 (30.6084, -15.6766)
  dimension "d366" = 1.2
  dimension "d367" = 1.2
  dimension "d368" = 1.2
  dimension "d369" = 34
  dimension "d371" = 1.2
  dimension "d372" = 1.2
  dimension "d373" = 1.2
  dimension "d376" = 360
  constraints: 448 end point, 12 parallel, 5 midpoint, 4 horizontal alignment, 4 point on line, 1 coincident, 1 horizontal, 1 vertical, 578 other
  measures "d366" distance between parallel lines of L4 L8
  measures "d367" distance between parallel lines of L11 L15
  measures "d368" distance between parallel lines of L20 L18
  measures "d369" vertical distance of point (52.459, -34.6) L22.end
  measures "d371" distance between parallel lines of L12 L33
  measures "d372" distance between parallel lines of L30 L45
  measures "d373" distance between parallel lines of L13 L39
extrude "Extrusion4" cut sketch "Sketch6" against normal through all
equation "\"d18\" = d15"
body "Solid1"
